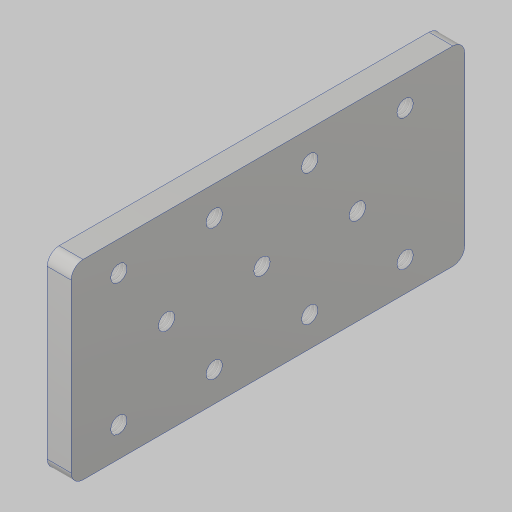
# Autodesk Inventor part: CL4-021
Saved by Autodesk Inventor 2023.5 (Build 275446000, 446)
## iProperties
Created: 2025-02-09
Part Number: CL4-021
Material: Aluminum 6061
Document SubType Name: Modeling
Designer: slick
Density: 2.7 g/cm^3
Appearance: Aluminum - Flat
Author: slick
Autodesk Inventor part; units mm, degrees
ref_plane "YZ Plane" through (0, 0, 0) normal (1, 0, 0) x (0, 1, 0)
ref_plane "XZ Plane" through (0, 0, 0) normal (0, 1, 0) x (-1, 0, 0)
ref_plane "XY Plane" through (0, 0, 0) normal (0, 0, 1) x (1, 0, 0)
sketch "Sketch1" plane through (0, 0, 0) normal (1, 0, 0) x (0, 1, 0)
  line L0 (-25.4, -52.3875) -> (25.4, -52.3875)
  line L1 (25.4, -52.3875) -> (25.4, 52.3875)
  line L2 (25.4, 52.3875) -> (-25.4, 52.3875)
  line L3 (-25.4, 52.3875) -> (-25.4, -52.3875)
  line L4 (-25.4, -52.3875) -> (25.4, 52.3875) construction
  line L5 (25.4, -52.3875) -> (-25.4, 52.3875) construction
  point P0 (0, 0)
  dimension "d0" = 104.775
  dimension "d1" = 50.8
  constraints: 12 end point, 2 midpoint, 2 parallel, 1 horizontal, 1 perpendicular
  measures "d0" distance of L0.end L1.end
  measures "d1" distance of L1.end L2.end
extrude "Extrusion1" add sketch "Sketch1" along normal blind 6.35
sketch "Sketch2" plane through (6.35, 0, 0) normal (1, 0, 0) x (0, 0, -1)
  line L0 (-39.6875, 17.4625) -> (-39.6875, -17.4625) construction
  line L1 (-52.3875, 25.4) -> (-52.3875, -25.4) construction
  line L2 (52.3875, 25.4) -> (52.3875, -25.4) construction
  line L3 (52.3875, -25.4) -> (-52.3875, -25.4) construction
  line L4 (-52.3875, -25.4) -> (-52.3875, 25.4) construction
  line L5 (-52.3875, 25.4) -> (52.3875, 25.4) construction
  point P0 (0, 0)
  point P1 (-26.9875, 0)
  point P2 (-39.6875, 0)
  point P3 (-52.3875, 0)
  point P4 (-14.2875, 17.4625)
  point P5 (-1.5875, 0)
  point P6 (-14.2875, -17.4625)
  point P7 (11.1125, 17.4625)
  point P8 (23.8125, 0)
  point P9 (11.1125, -17.4625)
  point P10 (36.5125, 17.4625)
  point P11 (49.2125, 0)
  point P12 (36.5125, -17.4625)
  dimension "d6" = 34.925
  dimension "d7" = 12.7
  dimension "d8" = 12.7
  dimension "d11" = 25.4
  constraints: 2 end point, 2 horizontal alignment, 2 midpoint, 1 horizontal, 1 vertical, 1 vertical alignment, 9 other
  measures "d6" distance of L0.start L0.end
  measures "d7" distance from line of L1 L0.start
  measures "d8" horizontal distance of point (-26.988, 0) L0.start
  measures "d11" distance of L0.start point (-14.288, 17.462)
hole "Hole1" at (6.35, -17.4625, 39.6875) at (6.35, 17.4625, 39.6875) at (6.35, 0, 26.9875) at (6.35, 17.4625, 14.2875) at (6.35, 0, 1.5875) at (6.35, -17.4625, 14.2875) at (6.35, 17.4625, -11.1125) at (6.35, 0, -23.8125) at (6.35, -17.4625, -11.1125) at (6.35, 17.4625, -36.5125) at (6.35, -17.4625, -36.5125) direction (-1, 0, 0) diameter 4.3434 end through all thread size "12-24 UNC" class "2B" standard "ANSI Unified Screw Threads"
fillet "Fillet1" radius 3.175 4 edges at (3.175, 25.4, 52.3875) (3.175, 25.4, -52.3875) (3.175, -25.4, -52.3875) (3.175, -25.4, 52.3875)
body "Solid1"
